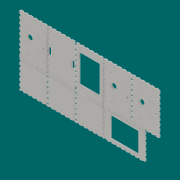
# Autodesk Inventor part: sheetA
Saved by Autodesk Inventor 2016 SP2 (Build 200236200, 236)
## iProperties
Created: 2016-09-27
Part Number: sheetA
Material: Generic
Document SubType Name: Modeling
Designer: sawaiz
Density: 1 g/cm^3
Appearance: Default
Author: sawaiz
Autodesk Inventor part; units mm, degrees
(part 1 of 3)
ref_plane "YZ Plane" through (0, 0, 0) normal (1, 0, 0) x (0, 1, 0)
ref_plane "XZ Plane" through (0, 0, 0) normal (0, 1, 0) x (-1, 0, 0)
sketch "Sketch1" plane through (0, 0, 0) normal (0, 0, 1) x (1, 0, 0)
  circle A0 centre (52.276, -59.1479) radius 1.078 projected
  circle A1 centre (17.276, -59.1479) radius 1.078 projected
  line L0 (43.815, -13.335) -> (40.005, -13.335) projected
  line L1 (40.005, -13.335) -> (40.005, -1.905) projected
  line L2 (40.005, -1.905) -> (43.815, -1.905) projected
  line L3 (43.815, -1.905) -> (43.815, -13.335) projected
  circle A2 centre (38.1, -15.24) radius 1.078 projected
  circle A3 centre (45.72, 0) radius 1.078 projected
  circle A4 centre (45.72, -15.24) radius 1.078 projected
  circle A5 centre (38.1, 0) radius 1.078 projected
  line L4 (54.825, -48.5) -> (56.825, -48.5) projected
  line L5 (56.825, -48.5) -> (56.825, -45) projected
  line L6 (56.825, -45) -> (60, -45) projected
  line L7 (60, -45) -> (60, -35) projected
  line L8 (60, -35) -> (56.825, -35) projected
  line L9 (56.825, -35) -> (56.825, -25) projected
  line L10 (56.825, -25) -> (60, -25) projected
  line L11 (60, -25) -> (60, -15) projected
  line L12 (60, -15) -> (56.825, -15) projected
  line L13 (56.825, -15) -> (56.825, -5) projected
  line L14 (56.825, -5) -> (60, -5) projected
  line L15 (60, -5) -> (60, 5) projected
  line L16 (60, 5) -> (56.825, 5) projected
  line L17 (56.825, 5) -> (56.825, 15) projected
  line L18 (56.825, 15) -> (60, 15) projected
  line L19 (60, 15) -> (60, 25) projected
  line L20 (60, 25) -> (56.825, 25) projected
  line L21 (56.825, 25) -> (56.825, 35) projected
  line L22 (56.825, 35) -> (60, 35) projected
  line L23 (60, 35) -> (60, 45) projected
  line L24 (60, 45) -> (56.825, 45) projected
  line L25 (56.825, 45) -> (56.825, 48.5) projected
  line L26 (56.825, 48.5) -> (54.825, 48.5) projected
  line L27 (54.825, 48.5) -> (54.825, 47.25) projected
  line L28 (54.825, 47.25) -> (52.325, 47.25) projected
  line L29 (52.325, 47.25) -> (52.325, 48.5) projected
  line L30 (52.325, 48.5) -> (46, 48.5) projected
  line L31 (46, 48.5) -> (46, 51.5) projected
  line L32 (46, 51.5) -> (52.325, 51.5) projected
  line L33 (52.325, 51.5) -> (52.325, 52.75) projected
  line L34 (52.325, 52.75) -> (54.825, 52.75) projected
  line L35 (54.825, 52.75) -> (54.825, 51.5) projected
  line L36 (54.825, 51.5) -> (56.825, 51.5) projected
  line L37 (56.825, 51.5) -> (56.825, 55) projected
  line L38 (56.825, 55) -> (60, 55) projected
  line L39 (60, 55) -> (60, 65) projected
  line L40 (60, 65) -> (56.825, 65) projected
  line L41 (56.825, 65) -> (56.825, 75) projected
  line L42 (56.825, 75) -> (60, 75) projected
  line L43 (60, 75) -> (60, 86.825) projected
  line L44 (55, 86.825) -> (60, 86.825) projected
  line L45 (55, 90) -> (55, 86.825) projected
  line L46 (45, 90) -> (55, 90) projected
  line L47 (45, 86.825) -> (45, 90) projected
  line L48 (45, 86.825) -> (35, 86.825) projected
  line L49 (35, 90) -> (35, 86.825) projected
  line L50 (25, 90) -> (35, 90) projected
  line L51 (25, 86.825) -> (25, 90) projected
  line L52 (25, 86.825) -> (15, 86.825) projected
  line L53 (15, 90) -> (15, 86.825) projected
  line L54 (5, 90) -> (15, 90) projected
  line L55 (5, 86.825) -> (5, 90) projected
  line L56 (5, 86.825) -> (-5, 86.825) projected
  line L57 (-5, 90) -> (-5, 86.825) projected
  line L58 (-15, 90) -> (-5, 90) projected
  line L59 (-15, 86.825) -> (-15, 90) projected
  line L60 (-15, 86.825) -> (-25, 86.825) projected
  line L61 (-25, 90) -> (-25, 86.825) projected
  line L62 (-35, 90) -> (-25, 90) projected
  line L63 (-35, 86.825) -> (-35, 90) projected
  line L64 (-35, 86.825) -> (-45, 86.825) projected
  line L65 (-45, 90) -> (-45, 86.825) projected
  line L66 (-55, 90) -> (-45, 90) projected
  line L67 (-55, 86.825) -> (-55, 90) projected
  line L68 (-55, 86.825) -> (-60, 86.825) projected
  line L69 (-60, 75) -> (-60, 86.825) projected
  line L70 (-56.825, 75) -> (-60, 75) projected
  line L71 (-56.825, 75) -> (-56.825, 65) projected
  line L72 (-60, 65) -> (-56.825, 65) projected
  line L73 (-60, 55) -> (-60, 65) projected
  line L74 (-56.825, 55) -> (-60, 55) projected
  line L75 (-56.825, 55) -> (-56.825, 45) projected
  line L76 (-60, 45) -> (-56.825, 45) projected
  line L77 (-60, 35) -> (-60, 45) projected
  line L78 (-56.825, 35) -> (-60, 35) projected
  line L79 (-56.825, 35) -> (-56.825, 25) projected
  line L80 (-60, 25) -> (-56.825, 25) projected
  line L81 (-60, 15) -> (-60, 25) projected
  line L82 (-56.825, 15) -> (-60, 15) projected
  line L83 (-56.825, 15) -> (-56.825, 5) projected
  line L84 (-60, 5) -> (-56.825, 5) projected
  line L85 (-60, -5) -> (-60, 5) projected
  line L86 (-56.825, -5) -> (-60, -5) projected
  line L87 (-56.825, -5) -> (-56.825, -15) projected
  line L88 (-60, -15) -> (-56.825, -15) projected
  line L89 (-60, -25) -> (-60, -15) projected
  line L90 (-56.825, -25) -> (-60, -25) projected
  line L91 (-56.825, -25) -> (-56.825, -35) projected
  line L92 (-60, -35) -> (-56.825, -35) projected
  line L93 (-60, -45) -> (-60, -35) projected
  line L94 (-56.825, -45) -> (-60, -45) projected
  line L95 (-56.825, -45) -> (-56.825, -55) projected
  line L96 (-60, -55) -> (-56.825, -55) projected
  line L97 (-60, -65) -> (-60, -55) projected
  line L98 (-56.825, -65) -> (-60, -65) projected
  line L99 (-56.825, -65) -> (-56.825, -75) projected
  line L100 (-60, -75) -> (-56.825, -75) projected
  line L101 (-60, -75) -> (-60, -86.825) projected
  line L102 (-60, -86.825) -> (-55, -86.825) projected
  line L103 (-55, -86.825) -> (-55, -90) projected
  line L104 (-55, -90) -> (-45, -90) projected
  line L105 (-45, -90) -> (-45, -86.825) projected
  line L106 (-45, -86.825) -> (-35, -86.825) projected
  line L107 (-35, -86.825) -> (-35, -90) projected
  line L108 (-35, -90) -> (-25, -90) projected
  line L109 (-25, -90) -> (-25, -86.825) projected
  line L110 (-25, -86.825) -> (-15, -86.825) projected
  line L111 (-15, -86.825) -> (-15, -90) projected
  line L112 (-15, -90) -> (-5, -90) projected
  line L113 (-5, -90) -> (-5, -86.825) projected
  line L114 (-5, -86.825) -> (5, -86.825) projected
  line L115 (5, -86.825) -> (5, -90) projected
  line L116 (5, -90) -> (15, -90) projected
  line L117 (15, -90) -> (15, -86.825) projected
  line L118 (15, -86.825) -> (25, -86.825) projected
  line L119 (25, -86.825) -> (25, -90) projected
  line L120 (25, -90) -> (35, -90) projected
  line L121 (35, -90) -> (35, -86.825) projected
  line L122 (35, -86.825) -> (45, -86.825) projected
  line L123 (45, -86.825) -> (45, -90) projected
  line L124 (45, -90) -> (55, -90) projected
  line L125 (55, -90) -> (55, -86.825) projected
  line L126 (55, -86.825) -> (60, -86.825) projected
  line L127 (60, -86.825) -> (60, -75) projected
  line L128 (60, -75) -> (56.825, -75) projected
  line L129 (56.825, -75) -> (56.825, -65) projected
  line L130 (56.825, -65) -> (60, -65) projected
  line L131 (60, -65) -> (60, -55) projected
  line L132 (60, -55) -> (56.825, -55) projected
  line L133 (56.825, -55) -> (56.825, -51.5) projected
  line L134 (56.825, -51.5) -> (54.825, -51.5) projected
  line L135 (54.825, -51.5) -> (54.825, -52.75) projected
  line L136 (54.825, -52.75) -> (52.325, -52.75) projected
  line L137 (52.325, -52.75) -> (52.325, -51.5) projected
  line L138 (52.325, -51.5) -> (46, -51.5) projected
  line L139 (46, -51.5) -> (46, -48.5) projected
  line L140 (46, -48.5) -> (52.325, -48.5) projected
  line L141 (52.325, -48.5) -> (52.325, -47.25) projected
  line L142 (52.325, -47.25) -> (54.825, -47.25) projected
  line L143 (54.825, -47.25) -> (54.825, -48.5) projected
  circle A6 centre (22.9972, -27.4451) radius 3 projected
  circle A7 centre (-22.9972, 54) radius 3 projected
  circle A8 centre (22.9972, 27.4451) radius 3 projected
  circle A9 centre (-22.9972, -54) radius 3 projected
  circle A10 centre (-15, 8.175) radius 11 projected
  line L144 (55, -207.185) -> (55, -210.36) projected
  line L145 (55, -210.36) -> (60, -210.36) projected
  line L146 (60, -210.36) -> (60, -205.36) projected
  line L147 (60, -205.36) -> (56.825, -205.36) projected
  line L148 (56.825, -205.36) -> (56.825, -195.36) projected
  line L149 (56.825, -195.36) -> (60, -195.36) projected
  line L150 (60, -195.36) -> (60, -185.36) projected
  line L151 (60, -185.36) -> (56.825, -185.36) projected
  line L152 (56.825, -185.36) -> (56.825, -175.36) projected
  line L153 (56.825, -175.36) -> (60, -175.36) projected
  line L154 (60, -175.36) -> (60, -165.36) projected
  line L155 (60, -165.36) -> (56.825, -165.36) projected
  line L156 (56.825, -165.36) -> (56.825, -155.36) projected
  line L157 (56.825, -155.36) -> (60, -155.36) projected
  line L158 (60, -155.36) -> (60, -145.36) projected
  line L159 (60, -145.36) -> (56.825, -145.36) projected
  line L160 (56.825, -145.36) -> (56.825, -135.36) projected
  line L161 (56.825, -135.36) -> (60, -135.36) projected
  line L162 (60, -135.36) -> (60, -125.36) projected
  line L163 (60, -125.36) -> (56.825, -125.36) projected
  line L164 (56.825, -125.36) -> (56.825, -115.36) projected
  line L165 (56.825, -115.36) -> (60, -115.36) projected
  line L166 (60, -115.36) -> (60, -105.36) projected
  line L167 (60, -105.36) -> (56.825, -105.36) projected
  line L168 (56.825, -105.36) -> (56.825, -95.36) projected
  line L169 (56.825, -95.36) -> (60, -95.36) projected
  line L170 (60, -95.36) -> (60, -90.36) projected
  line L171 (60, -90.36) -> (55, -90.36) projected
  line L172 (55, -90.36) -> (55, -93.535) projected
  line L173 (55, -93.535) -> (45, -93.535) projected
  line L174 (45, -93.535) -> (45, -90.36) projected
  line L175 (45, -90.36) -> (35, -90.36) projected
  line L176 (35, -90.36) -> (35, -93.535) projected
  line L177 (35, -93.535) -> (25, -93.535) projected
  line L178 (25, -93.535) -> (25, -90.36) projected
  line L179 (25, -90.36) -> (15, -90.36) projected
  line L180 (15, -90.36) -> (15, -93.535) projected
  line L181 (15, -93.535) -> (5, -93.535) projected
  line L182 (5, -93.535) -> (5, -90.36) projected
  line L183 (5, -90.36) -> (-5, -90.36) projected
  line L184 (-5, -90.36) -> (-5, -93.535) projected
  line L185 (-5, -93.535) -> (-15, -93.535) projected
  line L186 (-15, -93.535) -> (-15, -90.36) projected
  line L187 (-15, -90.36) -> (-25, -90.36) projected
  line L188 (-25, -90.36) -> (-25, -93.535) projected
  line L189 (-25, -93.535) -> (-35, -93.535) projected
  line L190 (-35, -93.535) -> (-35, -90.36) projected
  line L191 (-35, -90.36) -> (-45, -90.36) projected
  line L192 (-45, -90.36) -> (-45, -93.535) projected
  line L193 (-45, -93.535) -> (-55, -93.535) projected
  line L194 (-55, -93.535) -> (-55, -90.36) projected
  line L195 (-55, -90.36) -> (-60, -90.36) projected
  line L196 (-60, -90.36) -> (-60, -95.36) projected
  line L197 (-60, -95.36) -> (-56.825, -95.36) projected
  line L198 (-56.825, -95.36) -> (-56.825, -105.36) projected
  line L199 (-56.825, -105.36) -> (-60, -105.36) projected
  line L200 (-60, -105.36) -> (-60, -115.36) projected
  line L201 (-60, -115.36) -> (-56.825, -115.36) projected
  line L202 (-56.825, -115.36) -> (-56.825, -125.36) projected
  line L203 (-56.825, -125.36) -> (-60, -125.36) projected
  line L204 (-60, -125.36) -> (-60, -135.36) projected
  line L205 (-60, -135.36) -> (-56.825, -135.36) projected
  line L206 (-56.825, -135.36) -> (-56.825, -145.36) projected
  line L207 (-56.825, -145.36) -> (-60, -145.36) projected
  line L208 (-60, -145.36) -> (-60, -155.36) projected
  line L209 (-60, -155.36) -> (-56.825, -155.36) projected
  line L210 (-56.825, -155.36) -> (-56.825, -165.36) projected
  line L211 (-56.825, -165.36) -> (-60, -165.36) projected
  line L212 (-60, -165.36) -> (-60, -175.36) projected
  line L213 (-60, -175.36) -> (-56.825, -175.36) projected
  line L214 (-56.825, -175.36) -> (-56.825, -185.36) projected
  line L215 (-56.825, -185.36) -> (-60, -185.36) projected
  line L216 (-60, -185.36) -> (-60, -195.36) projected
  line L217 (-60, -195.36) -> (-56.825, -195.36) projected
  line L218 (-56.825, -195.36) -> (-56.825, -205.36) projected
  line L219 (-56.825, -205.36) -> (-60, -205.36) projected
  line L220 (-60, -205.36) -> (-60, -210.36) projected
  line L221 (-60, -210.36) -> (-55, -210.36) projected
  line L222 (-55, -210.36) -> (-55, -207.185) projected
  line L223 (-55, -207.185) -> (-45, -207.185) projected
  line L224 (-45, -207.185) -> (-45, -210.36) projected
  line L225 (-45, -210.36) -> (-35, -210.36) projected
  line L226 (-35, -210.36) -> (-35, -207.185) projected
  line L227 (-35, -207.185) -> (-25, -207.185) projected
  line L228 (-25, -207.185) -> (-25, -210.36) projected
  line L229 (-25, -210.36) -> (-15, -210.36) projected
  line L230 (-15, -210.36) -> (-15, -207.185) projected
  line L231 (-15, -207.185) -> (-5, -207.185) projected
  line L232 (-5, -207.185) -> (-5, -210.36) projected
  line L233 (-5, -210.36) -> (5, -210.36) projected
  line L234 (5, -210.36) -> (5, -207.185) projected
  line L235 (5, -207.185) -> (15, -207.185) projected
  line L236 (15, -207.185) -> (15, -210.36) projected
  line L237 (15, -210.36) -> (25, -210.36) projected
  line L238 (25, -210.36) -> (25, -207.185) projected
  line L239 (25, -207.185) -> (35, -207.185) projected
  line L240 (35, -207.185) -> (35, -210.36) projected
  line L241 (35, -210.36) -> (45, -210.36) projected
  line L242 (45, -210.36) -> (45, -207.185) projected
  line L243 (45, -207.185) -> (55, -207.185) projected
  line L244 (175.36, -207.185) -> (175.36, -210.36) projected
  line L245 (175.36, -210.36) -> (180.36, -210.36) projected
  line L246 (180.36, -210.36) -> (180.36, -205.36) projected
  line L247 (180.36, -205.36) -> (177.185, -205.36) projected
  line L248 (177.185, -205.36) -> (177.185, -195.36) projected
  line L249 (177.185, -195.36) -> (180.36, -195.36) projected
  line L250 (180.36, -195.36) -> (180.36, -185.36) projected
  line L251 (180.36, -185.36) -> (177.185, -185.36) projected
  line L252 (177.185, -185.36) -> (177.185, -175.36) projected
  line L253 (177.185, -175.36) -> (180.36, -175.36) projected
  line L254 (180.36, -175.36) -> (180.36, -165.36) projected
  line L255 (180.36, -165.36) -> (177.185, -165.36) projected
  line L256 (177.185, -165.36) -> (177.185, -155.36) projected
  line L257 (177.185, -155.36) -> (180.36, -155.36) projected
  line L258 (180.36, -155.36) -> (180.36, -145.36) projected
  line L259 (180.36, -145.36) -> (177.185, -145.36) projected
  line L260 (177.185, -145.36) -> (177.185, -135.36) projected
  line L261 (177.185, -135.36) -> (180.36, -135.36) projected
  line L262 (180.36, -135.36) -> (180.36, -125.36) projected
  line L263 (180.36, -125.36) -> (177.185, -125.36) projected
  line L264 (177.185, -125.36) -> (177.185, -115.36) projected
  line L265 (177.185, -115.36) -> (180.36, -115.36) projected
  line L266 (180.36, -115.36) -> (180.36, -105.36) projected
  line L267 (180.36, -105.36) -> (177.185, -105.36) projected
  line L268 (177.185, -105.36) -> (177.185, -95.36) projected
  line L269 (177.185, -95.36) -> (180.36, -95.36) projected
  line L270 (180.36, -95.36) -> (180.36, -90.36) projected
  line L271 (180.36, -90.36) -> (175.36, -90.36) projected
  line L272 (175.36, -90.36) -> (175.36, -93.535) projected
  line L273 (175.36, -93.535) -> (165.36, -93.535) projected
  line L274 (165.36, -93.535) -> (165.36, -90.36) projected
  line L275 (165.36, -90.36) -> (155.36, -90.36) projected
  line L276 (155.36, -90.36) -> (155.36, -93.535) projected
  line L277 (155.36, -93.535) -> (145.36, -93.535) projected
  line L278 (145.36, -93.535) -> (145.36, -90.36) projected
  line L279 (145.36, -90.36) -> (135.36, -90.36) projected
  line L280 (135.36, -90.36) -> (135.36, -93.535) projected
  line L281 (135.36, -93.535) -> (125.36, -93.535) projected
  line L282 (125.36, -93.535) -> (125.36, -90.36) projected
  line L283 (125.36, -90.36) -> (115.36, -90.36) projected
  line L284 (115.36, -90.36) -> (115.36, -93.535) projected
  line L285 (115.36, -93.535) -> (105.36, -93.535) projected
  line L286 (105.36, -93.535) -> (105.36, -90.36) projected
  line L287 (105.36, -90.36) -> (95.36, -90.36) projected
  line L288 (95.36, -90.36) -> (95.36, -93.535) projected
  line L289 (95.36, -93.535) -> (85.36, -93.535) projected
  line L290 (85.36, -93.535) -> (85.36, -90.36) projected
  line L291 (85.36, -90.36) -> (75.36, -90.36) projected
  line L292 (75.36, -90.36) -> (75.36, -93.535) projected
  line L293 (75.36, -93.535) -> (65.36, -93.535) projected
  line L294 (65.36, -93.535) -> (65.36, -90.36) projected
  line L295 (65.36, -90.36) -> (60.36, -90.36) projected
  line L296 (60.36, -90.36) -> (60.36, -95.36) projected
  line L297 (60.36, -95.36) -> (63.535, -95.36) projected
  line L298 (63.535, -95.36) -> (63.535, -105.36) projected
  line L299 (63.535, -105.36) -> (60.36, -105.36) projected
  line L300 (60.36, -105.36) -> (60.36, -115.36) projected
  line L301 (60.36, -115.36) -> (63.535, -115.36) projected
  line L302 (63.535, -115.36) -> (63.535, -125.36) projected
  line L303 (63.535, -125.36) -> (60.36, -125.36) projected
  line L304 (60.36, -125.36) -> (60.36, -135.36) projected
  line L305 (60.36, -135.36) -> (63.535, -135.36) projected
  line L306 (63.535, -135.36) -> (63.535, -145.36) projected
  line L307 (63.535, -145.36) -> (60.36, -145.36) projected
  line L308 (60.36, -145.36) -> (60.36, -155.36) projected
  line L309 (60.36, -155.36) -> (63.535, -155.36) projected
  line L310 (63.535, -155.36) -> (63.535, -165.36) projected
  line L311 (63.535, -165.36) -> (60.36, -165.36) projected
  line L312 (60.36, -165.36) -> (60.36, -175.36) projected
  line L313 (60.36, -175.36) -> (63.535, -175.36) projected
  line L314 (63.535, -175.36) -> (63.535, -185.36) projected
  line L315 (63.535, -185.36) -> (60.36, -185.36) projected
  line L316 (60.36, -185.36) -> (60.36, -195.36) projected
  line L317 (60.36, -195.36) -> (63.535, -195.36) projected
  line L318 (63.535, -195.36) -> (63.535, -205.36) projected
  line L319 (63.535, -205.36) -> (60.36, -205.36) projected
  line L320 (60.36, -205.36) -> (60.36, -210.36) projected
  line L321 (60.36, -210.36) -> (65.36, -210.36) projected
  line L322 (65.36, -210.36) -> (65.36, -207.185) projected
  line L323 (65.36, -207.185) -> (75.36, -207.185) projected
  line L324 (75.36, -207.185) -> (75.36, -210.36) projected
  line L325 (75.36, -210.36) -> (85.36, -210.36) projected
  line L326 (85.36, -210.36) -> (85.36, -207.185) projected
  line L327 (85.36, -207.185) -> (95.36, -207.185) projected
  line L328 (95.36, -207.185) -> (95.36, -210.36) projected
  line L329 (95.36, -210.36) -> (105.36, -210.36) projected
  line L330 (105.36, -210.36) -> (105.36, -207.185) projected
  line L331 (105.36, -207.185) -> (115.36, -207.185) projected
  line L332 (115.36, -207.185) -> (115.36, -210.36) projected
  line L333 (115.36, -210.36) -> (125.36, -210.36) projected
  line L334 (125.36, -210.36) -> (125.36, -207.185) projected
  line L335 (125.36, -207.185) -> (135.36, -207.185) projected
  line L336 (135.36, -207.185) -> (135.36, -210.36) projected
  line L337 (135.36, -210.36) -> (145.36, -210.36) projected
  line L338 (145.36, -210.36) -> (145.36, -207.185) projected
  line L339 (145.36, -207.185) -> (155.36, -207.185) projected
  line L340 (155.36, -207.185) -> (155.36, -210.36) projected
  line L341 (155.36, -210.36) -> (165.36, -210.36) projected
  line L342 (165.36, -210.36) -> (165.36, -207.185) projected
  line L343 (165.36, -207.185) -> (175.36, -207.185) projected
  line L344 (165.36, -15) -> (165.36, 15) projected
  line L345 (165.36, 15) -> (175.36, 15) projected
  line L346 (175.36, 15) -> (175.36, -15) projected
  line L347 (175.36, -15) -> (165.36, -15) projected
  line L348 (65.36, -15) -> (65.36, 15) projected
  line L349 (65.36, 15) -> (75.36, 15) projected
  line L350 (75.36, 15) -> (75.36, -15) projected
  line L351 (75.36, -15) -> (65.36, -15) projected
  circle A11 centre (177.185, -50) radius 1.7 projected
  circle A12 centre (177.185, 50) radius 1.7 projected
  circle A13 centre (63.535, -50) radius 1.7 projected
  circle A14 centre (63.535, 50) radius 1.7 projected
  line L352 (177.185, 75) -> (177.185, 86.825) projected
  line L353 (177.185, 86.825) -> (175.36, 86.825) projected
  line L354 (175.36, 86.825) -> (175.36, 90) projected
  line L355 (175.36, 90) -> (165.36, 90) projected
  line L356 (165.36, 90) -> (165.36, 86.825) projected
  line L357 (165.36, 86.825) -> (155.36, 86.825) projected
  line L358 (155.36, 86.825) -> (155.36, 90) projected
  line L359 (155.36, 90) -> (145.36, 90) projected
  line L360 (145.36, 90) -> (145.36, 86.825) projected
  line L361 (145.36, 86.825) -> (135.36, 86.825) projected
  line L362 (135.36, 86.825) -> (135.36, 90) projected
  line L363 (135.36, 90) -> (125.36, 90) projected
  line L364 (125.36, 90) -> (125.36, 86.825) projected
  line L365 (125.36, 86.825) -> (115.36, 86.825) projected
  line L366 (115.36, 86.825) -> (115.36, 90) projected
  line L367 (115.36, 90) -> (105.36, 90) projected
  line L368 (105.36, 90) -> (105.36, 86.825) projected
  line L369 (105.36, 86.825) -> (95.36, 86.825) projected
  line L370 (95.36, 86.825) -> (95.36, 90) projected
  line L371 (95.36, 90) -> (85.36, 90) projected
  line L372 (85.36, 90) -> (85.36, 86.825) projected
  line L373 (85.36, 86.825) -> (75.36, 86.825) projected
  line L374 (75.36, 86.825) -> (75.36, 90) projected
  line L375 (75.36, 90) -> (65.36, 90) projected
  line L376 (65.36, 90) -> (65.36, 86.825) projected
  line L377 (65.36, 86.825) -> (63.535, 86.825) projected
  line L378 (63.535, 86.825) -> (63.535, 75) projected
  line L379 (63.535, 75) -> (60.36, 75) projected
  line L380 (60.36, 75) -> (60.36, 65) projected
  line L381 (60.36, 65) -> (63.535, 65) projected
  line L382 (63.535, 65) -> (63.535, 55) projected
  line L383 (63.535, 55) -> (60.36, 55) projected
  line L384 (60.36, 55) -> (60.36, 45) projected
  line L385 (60.36, 45) -> (63.535, 45) projected
  line L386 (63.535, 45) -> (63.535, 35) projected
  line L387 (63.535, 35) -> (60.36, 35) projected
  line L388 (60.36, 35) -> (60.36, 25) projected
  line L389 (60.36, 25) -> (63.535, 25) projected
  line L390 (63.535, 25) -> (63.535, 15) projected
  line L391 (63.535, 15) -> (60.36, 15) projected
  line L392 (60.36, 15) -> (60.36, 5) projected
  line L393 (60.36, 5) -> (63.535, 5) projected
  line L394 (63.535, 5) -> (63.535, -5) projected
  line L395 (63.535, -5) -> (60.36, -5) projected
  line L396 (60.36, -5) -> (60.36, -15) projected
  line L397 (60.36, -15) -> (63.535, -15) projected
  line L398 (63.535, -15) -> (63.535, -25) projected
  line L399 (63.535, -25) -> (60.36, -25) projected
  line L400 (60.36, -25) -> (60.36, -35) projected
  line L401 (60.36, -35) -> (63.535, -35) projected
  line L402 (63.535, -35) -> (63.535, -45) projected
  line L403 (63.535, -45) -> (60.36, -45) projected
  line L404 (60.36, -45) -> (60.36, -55) projected
  line L405 (60.36, -55) -> (63.535, -55) projected
  line L406 (63.535, -55) -> (63.535, -65) projected
  line L407 (63.535, -65) -> (60.36, -65) projected
  line L408 (60.36, -65) -> (60.36, -75) projected
  line L409 (60.36, -75) -> (63.535, -75) projected
  line L410 (63.535, -75) -> (63.535, -86.825) projected
  line L411 (63.535, -86.825) -> (65.36, -86.825) projected
  line L412 (65.36, -86.825) -> (65.36, -90) projected
  line L413 (65.36, -90) -> (75.36, -90) projected
  line L414 (75.36, -90) -> (75.36, -86.825) projected
  line L415 (75.36, -86.825) -> (85.36, -86.825) projected
  line L416 (85.36, -86.825) -> (85.36, -90) projected
  line L417 (85.36, -90) -> (95.36, -90) projected
  line L418 (95.36, -90) -> (95.36, -86.825) projected
  line L419 (95.36, -86.825) -> (105.36, -86.825) projected
  line L420 (105.36, -86.825) -> (105.36, -90) projected
  line L421 (105.36, -90) -> (115.36, -90) projected
  line L422 (115.36, -90) -> (115.36, -86.825) projected
  line L423 (115.36, -86.825) -> (125.36, -86.825) projected
  line L424 (125.36, -86.825) -> (125.36, -90) projected
  line L425 (125.36, -90) -> (135.36, -90) projected
  line L426 (135.36, -90) -> (135.36, -86.825) projected
  line L427 (135.36, -86.825) -> (145.36, -86.825) projected
  line L428 (145.36, -86.825) -> (145.36, -90) projected
  line L429 (145.36, -90) -> (155.36, -90) projected
  line L430 (155.36, -90) -> (155.36, -86.825) projected
  line L431 (155.36, -86.825) -> (165.36, -86.825) projected
  line L432 (165.36, -86.825) -> (165.36, -90) projected
  line L433 (165.36, -90) -> (175.36, -90) projected
  line L434 (175.36, -90) -> (175.36, -86.825) projected
  line L435 (175.36, -86.825) -> (177.185, -86.825) projected
  line L436 (177.185, -86.825) -> (177.185, -75) projected
  line L437 (177.185, -75) -> (180.36, -75) projected
  line L438 (180.36, -75) -> (180.36, -65) projected
  line L439 (180.36, -65) -> (177.185, -65) projected
  line L440 (177.185, -65) -> (177.185, -55) projected
  line L441 (177.185, -55) -> (180.36, -55) projected
  line L442 (180.36, -55) -> (180.36, -45) projected
  line L443 (180.36, -45) -> (177.185, -45) projected
  line L444 (177.185, -45) -> (177.185, -35) projected
  line L445 (177.185, -35) -> (180.36, -35) projected
  line L446 (180.36, -35) -> (180.36, -25) projected
  line L447 (180.36, -25) -> (177.185, -25) projected
  line L448 (177.185, -25) -> (177.185, -15) projected
  line L449 (177.185, -15) -> (180.36, -15) projected
  line L450 (180.36, -15) -> (180.36, -5) projected
  line L451 (180.36, -5) -> (177.185, -5) projected
  line L452 (177.185, -5) -> (177.185, 5) projected
  line L453 (177.185, 5) -> (180.36, 5) projected
  line L454 (180.36, 5) -> (180.36, 15) projected
  line L455 (180.36, 15) -> (177.185, 15) projected
  line L456 (177.185, 15) -> (177.185, 25) projected
  line L457 (177.185, 25) -> (180.36, 25) projected
  line L458 (180.36, 25) -> (180.36, 35) projected
  line L459 (180.36, 35) -> (177.185, 35) projected
  line L460 (177.185, 35) -> (177.185, 45) projected
  line L461 (177.185, 45) -> (180.36, 45) projected
  line L462 (180.36, 45) -> (180.36, 55) projected
  line L463 (180.36, 55) -> (177.185, 55) projected
  line L464 (177.185, 55) -> (177.185, 65) projected
  line L465 (177.185, 65) -> (180.36, 65) projected
  line L466 (180.36, 65) -> (180.36, 75) projected
  line L467 (180.36, 75) -> (177.185, 75) projected
  line L468 (295.72, -207.185) -> (295.72, -210.36) projected
  line L469 (295.72, -210.36) -> (300.72, -210.36) projected
  line L470 (300.72, -210.36) -> (300.72, -205.36) projected
  line L471 (300.72, -205.36) -> (297.545, -205.36) projected
  line L472 (297.545, -205.36) -> (297.545, -195.36) projected
  line L473 (297.545, -195.36) -> (300.72, -195.36) projected
  line L474 (300.72, -195.36) -> (300.72, -185.36) projected
  line L475 (300.72, -185.36) -> (297.545, -185.36) projected
  line L476 (297.545, -185.36) -> (297.545, -175.36) projected
  line L477 (297.545, -175.36) -> (300.72, -175.36) projected
  line L478 (300.72, -175.36) -> (300.72, -165.36) projected
  line L479 (300.72, -165.36) -> (297.545, -165.36) projected
  line L480 (297.545, -165.36) -> (297.545, -155.36) projected
  line L481 (297.545, -155.36) -> (300.72, -155.36) projected
  line L482 (300.72, -155.36) -> (300.72, -145.36) projected
  line L483 (300.72, -145.36) -> (297.545, -145.36) projected
  line L484 (297.545, -145.36) -> (297.545, -135.36) projected
  line L485 (297.545, -135.36) -> (300.72, -135.36) projected
  line L486 (300.72, -135.36) -> (300.72, -125.36) projected
  line L487 (300.72, -125.36) -> (297.545, -125.36) projected
  line L488 (297.545, -125.36) -> (297.545, -115.36) projected
  line L489 (297.545, -115.36) -> (300.72, -115.36) projected
  line L490 (300.72, -115.36) -> (300.72, -105.36) projected
  line L491 (300.72, -105.36) -> (297.545, -105.36) projected
  line L492 (297.545, -105.36) -> (297.545, -95.36) projected
  line L493 (297.545, -95.36) -> (300.72, -95.36) projected
  line L494 (300.72, -95.36) -> (300.72, -90.36) projected
  line L495 (300.72, -90.36) -> (295.72, -90.36) projected
  line L496 (295.72, -90.36) -> (295.72, -93.535) projected
  line L497 (295.72, -93.535) -> (285.72, -93.535) projected
  line L498 (285.72, -93.535) -> (285.72, -90.36) projected
  line L499 (285.72, -90.36) -> (275.72, -90.36) projected
  line L500 (275.72, -90.36) -> (275.72, -93.535) projected
  line L501 (275.72, -93.535) -> (265.72, -93.535) projected
  line L502 (265.72, -93.535) -> (265.72, -90.36) projected
  line L503 (265.72, -90.36) -> (255.72, -90.36) projected
  line L504 (255.72, -90.36) -> (255.72, -93.535) projected
  line L505 (255.72, -93.535) -> (245.72, -93.535) projected
  line L506 (245.72, -93.535) -> (245.72, -90.36) projected
  line L507 (245.72, -90.36) -> (235.72, -90.36) projected
  line L508 (235.72, -90.36) -> (235.72, -93.535) projected
  line L509 (235.72, -93.535) -> (225.72, -93.535) projected
  line L510 (225.72, -93.535) -> (225.72, -90.36) projected
  line L511 (225.72, -90.36) -> (215.72, -90.36) projected
  line L512 (215.72, -90.36) -> (215.72, -93.535) projected
  line L513 (215.72, -93.535) -> (205.72, -93.535) projected
  line L514 (205.72, -93.535) -> (205.72, -90.36) projected
  line L515 (205.72, -90.36) -> (195.72, -90.36) projected
  line L516 (195.72, -90.36) -> (195.72, -93.535) projected
  line L517 (195.72, -93.535) -> (185.72, -93.535) projected
  line L518 (185.72, -93.535) -> (185.72, -90.36) projected
  line L519 (185.72, -90.36) -> (180.72, -90.36) projected
  line L520 (180.72, -90.36) -> (180.72, -95.36) projected
  line L521 (180.72, -95.36) -> (183.895, -95.36) projected
  line L522 (183.895, -95.36) -> (183.895, -105.36) projected
  line L523 (183.895, -105.36) -> (180.72, -105.36) projected
  line L524 (180.72, -105.36) -> (180.72, -115.36) projected
  line L525 (180.72, -115.36) -> (183.895, -115.36) projected
  line L526 (183.895, -115.36) -> (183.895, -125.36) projected
  line L527 (183.895, -125.36) -> (180.72, -125.36) projected
  line L528 (180.72, -125.36) -> (180.72, -135.36) projected
  line L529 (180.72, -135.36) -> (183.895, -135.36) projected
  line L530 (183.895, -135.36) -> (183.895, -145.36) projected
  line L531 (183.895, -145.36) -> (180.72, -145.36) projected
  line L532 (180.72, -145.36) -> (180.72, -155.36) projected
  line L533 (180.72, -155.36) -> (183.895, -155.36) projected
  line L534 (183.895, -155.36) -> (183.895, -165.36) projected
  line L535 (183.895, -165.36) -> (180.72, -165.36) projected
  line L536 (180.72, -165.36) -> (180.72, -175.36) projected
  line L537 (180.72, -175.36) -> (183.895, -175.36) projected
  line L538 (183.895, -175.36) -> (183.895, -185.36) projected
  line L539 (183.895, -185.36) -> (180.72, -185.36) projected
  line L540 (180.72, -185.36) -> (180.72, -195.36) projected
  line L541 (180.72, -195.36) -> (183.895, -195.36) projected
  line L542 (183.895, -195.36) -> (183.895, -205.36) projected
  line L543 (183.895, -205.36) -> (180.72, -205.36) projected
  line L544 (180.72, -205.36) -> (180.72, -210.36) projected
  line L545 (180.72, -210.36) -> (185.72, -210.36) projected
  line L546 (185.72, -210.36) -> (185.72, -207.185) projected
  line L547 (185.72, -207.185) -> (195.72, -207.185) projected
  line L548 (195.72, -207.185) -> (195.72, -210.36) projected
  line L549 (195.72, -210.36) -> (205.72, -210.36) projected
  line L550 (205.72, -210.36) -> (205.72, -207.185) projected
  line L551 (205.72, -207.185) -> (215.72, -207.185) projected
  line L552 (215.72, -207.185) -> (215.72, -210.36) projected
  line L553 (215.72, -210.36) -> (225.72, -210.36) projected
  line L554 (225.72, -210.36) -> (225.72, -207.185) projected
  line L555 (225.72, -207.185) -> (235.72, -207.185) projected
  line L556 (235.72, -207.185) -> (235.72, -210.36) projected
  line L557 (235.72, -210.36) -> (245.72, -210.36) projected
  line L558 (245.72, -210.36) -> (245.72, -207.185) projected
  line L559 (245.72, -207.185) -> (255.72, -207.185) projected
  line L560 (255.72, -207.185) -> (255.72, -210.36) projected
  line L561 (255.72, -210.36) -> (265.72, -210.36) projected
  line L562 (265.72, -210.36) -> (265.72, -207.185) projected
  line L563 (265.72, -207.185) -> (275.72, -207.185) projected
  line L564 (275.72, -207.185) -> (275.72, -210.36) projected
  line L565 (275.72, -210.36) -> (285.72, -210.36) projected
  line L566 (285.72, -210.36) -> (285.72, -207.185) projected
  line L567 (285.72, -207.185) -> (295.72, -207.185) projected
  line L568 (297.545, 75) -> (297.545, 86.825) projected
  line L569 (297.545, 86.825) -> (295.72, 86.825) projected
  line L570 (295.72, 86.825) -> (295.72, 90) projected
  line L571 (295.72, 90) -> (285.72, 90) projected
  line L572 (285.72, 90) -> (285.72, 86.825) projected
  line L573 (285.72, 86.825) -> (275.72, 86.825) projected
  line L574 (275.72, 86.825) -> (275.72, 90) projected
  line L575 (275.72, 90) -> (265.72, 90) projected
  line L576 (265.72, 90) -> (265.72, 86.825) projected
  line L577 (265.72, 86.825) -> (255.72, 86.825) projected
  line L578 (255.72, 86.825) -> (255.72, 90) projected
  line L579 (255.72, 90) -> (245.72, 90) projected
  line L580 (245.72, 90) -> (245.72, 86.825) projected
  line L581 (245.72, 86.825) -> (235.72, 86.825) projected
  line L582 (235.72, 86.825) -> (235.72, 90) projected
  line L583 (235.72, 90) -> (225.72, 90) projected
  line L584 (225.72, 90) -> (225.72, 86.825) projected
  line L585 (225.72, 86.825) -> (215.72, 86.825) projected
  line L586 (215.72, 86.825) -> (215.72, 90) projected
  line L587 (215.72, 90) -> (205.72, 90) projected
  line L588 (205.72, 90) -> (205.72, 86.825) projected
  line L589 (205.72, 86.825) -> (195.72, 86.825) projected
  line L590 (195.72, 86.825) -> (195.72, 90) projected
  line L591 (195.72, 90) -> (185.72, 90) projected
  line L592 (185.72, 90) -> (185.72, 86.825) projected
  line L593 (185.72, 86.825) -> (183.895, 86.825) projected
  line L594 (183.895, 86.825) -> (183.895, 75) projected
  line L595 (183.895, 75) -> (180.72, 75) projected
  line L596 (180.72, 75) -> (180.72, 65) projected
  line L597 (180.72, 65) -> (183.895, 65) projected
  line L598 (183.895, 65) -> (183.895, 55) projected
  line L599 (183.895, 55) -> (180.72, 55) projected
  line L600 (180.72, 55) -> (180.72, 45) projected
  line L601 (180.72, 45) -> (183.895, 45) projected
  line L602 (183.895, 45) -> (183.895, 35) projected
  line L603 (183.895, 35) -> (180.72, 35) projected
  line L604 (180.72, 35) -> (180.72, 25) projected
  line L605 (180.72, 25) -> (183.895, 25) projected
  line L606 (183.895, 25) -> (183.895, 15) projected
  line L607 (183.895, 15) -> (180.72, 15) projected
  line L608 (180.72, 15) -> (180.72, 5) projected
  line L609 (180.72, 5) -> (183.895, 5) projected
  line L610 (183.895, 5) -> (183.895, -5) projected
  line L611 (183.895, -5) -> (180.72, -5) projected
  line L612 (180.72, -5) -> (180.72, -15) projected
  line L613 (180.72, -15) -> (183.895, -15) projected
  line L614 (183.895, -15) -> (183.895, -25) projected
  line L615 (183.895, -25) -> (180.72, -25) projected
  line L616 (180.72, -25) -> (180.72, -35) projected
  line L617 (180.72, -35) -> (183.895, -35) projected
  line L618 (183.895, -35) -> (183.895, -45) projected
  line L619 (183.895, -45) -> (180.72, -45) projected
  line L620 (180.72, -45) -> (180.72, -55) projected
  line L621 (180.72, -55) -> (183.895, -55) projected
  line L622 (183.895, -55) -> (183.895, -65) projected
  line L623 (183.895, -65) -> (180.72, -65) projected
  line L624 (180.72, -65) -> (180.72, -75) projected
  line L625 (180.72, -75) -> (183.895, -75) projected
  line L626 (183.895, -75) -> (183.895, -86.825) projected
  line L627 (183.895, -86.825) -> (185.72, -86.825) projected
  line L628 (185.72, -86.825) -> (185.72, -90) projected
  line L629 (185.72, -90) -> (195.72, -90) projected
  line L630 (195.72, -90) -> (195.72, -86.825) projected
  line L631 (195.72, -86.825) -> (205.72, -86.825) projected
  line L632 (205.72, -86.825) -> (205.72, -90) projected
  line L633 (205.72, -90) -> (215.72, -90) projected
  line L634 (215.72, -90) -> (215.72, -86.825) projected
  line L635 (215.72, -86.825) -> (225.72, -86.825) projected
  line L636 (225.72, -86.825) -> (225.72, -90) projected
  line L637 (225.72, -90) -> (235.72, -90) projected
  line L638 (235.72, -90) -> (235.72, -86.825) projected
  line L639 (235.72, -86.825) -> (245.72, -86.825) projected
  line L640 (245.72, -86.825) -> (245.72, -90) projected
  line L641 (245.72, -90) -> (255.72, -90) projected
  line L642 (255.72, -90) -> (255.72, -86.825) projected
  line L643 (255.72, -86.825) -> (265.72, -86.825) projected
  line L644 (265.72, -86.825) -> (265.72, -90) projected
  line L645 (265.72, -90) -> (275.72, -90) projected
  line L646 (275.72, -90) -> (275.72, -86.825) projected
  line L647 (275.72, -86.825) -> (285.72, -86.825) projected
  line L648 (285.72, -86.825) -> (285.72, -90) projected
  line L649 (285.72, -90) -> (295.72, -90) projected
  line L650 (295.72, -90) -> (295.72, -86.825) projected
  line L651 (295.72, -86.825) -> (297.545, -86.825) projected
  line L652 (297.545, -86.825) -> (297.545, -75) projected
  line L653 (297.545, -75) -> (300.72, -75) projected
  line L654 (300.72, -75) -> (300.72, -65) projected
  line L655 (300.72, -65) -> (297.545, -65) projected
  line L656 (297.545, -65) -> (297.545, -55) projected
  line L657 (297.545, -55) -> (300.72, -55) projected
  line L658 (300.72, -55) -> (300.72, -45) projected
  line L659 (300.72, -45) -> (297.545, -45) projected
  line L660 (297.545, -45) -> (297.545, -35) projected
  line L661 (297.545, -35) -> (300.72, -35) projected
  line L662 (300.72, -35) -> (300.72, -25) projected
  line L663 (300.72, -25) -> (297.545, -25) projected
  line L664 (297.545, -25) -> (297.545, -15) projected
  line L665 (297.545, -15) -> (300.72, -15) projected
  line L666 (300.72, -15) -> (300.72, -5) projected
  line L667 (300.72, -5) -> (297.545, -5) projected
  line L668 (297.545, -5) -> (297.545, 5) projected
  line L669 (297.545, 5) -> (300.72, 5) projected
  line L670 (300.72, 5) -> (300.72, 15) projected
  line L671 (300.72, 15) -> (297.545, 15) projected
  line L672 (297.545, 15) -> (297.545, 25) projected
  line L673 (297.545, 25) -> (300.72, 25) projected
  line L674 (300.72, 25) -> (300.72, 35) projected
  line L675 (300.72, 35) -> (297.545, 35) projected
  line L676 (297.545, 35) -> (297.545, 45) projected
  line L677 (297.545, 45) -> (300.72, 45) projected
  line L678 (300.72, 45) -> (300.72, 55) projected
  line L679 (300.72, 55) -> (297.545, 55) projected
  line L680 (297.545, 55) -> (297.545, 65) projected
  line L681 (297.545, 65) -> (300.72, 65) projected
  line L682 (300.72, 65) -> (300.72, 75) projected
  line L683 (300.72, 75) -> (297.545, 75) projected
  line L684 (196.92, -60) -> (196.92, 60) projected
  line L685 (196.92, 60) -> (284.52, 60) projected
  line L686 (284.52, 60) -> (284.52, -60) projected
  line L687 (284.52, -60) -> (196.92, -60) projected
  line L688 (404.895, -13.335) -> (401.085, -13.335) projected
  line L689 (401.085, -13.335) -> (401.085, -1.905) projected
  line L690 (401.085, -1.905) -> (404.895, -1.905) projected
  line L691 (404.895, -1.905) -> (404.895, -13.335) projected
  circle A15 centre (399.18, -15.24) radius 1.078 projected
  circle A16 centre (406.8, 0) radius 1.078 projected
  circle A17 centre (406.8, -15.24) radius 1.078 projected
  circle A18 centre (399.18, 0) radius 1.078 projected
  line L692 (415.905, -48.5) -> (417.905, -48.5) projected
  line L693 (417.905, -48.5) -> (417.905, -45) projected
  line L694 (417.905, -45) -> (421.08, -45) projected
  line L695 (421.08, -45) -> (421.08, -35) projected
  line L696 (421.08, -35) -> (417.905, -35) projected
  line L697 (417.905, -35) -> (417.905, -25) projected
  line L698 (417.905, -25) -> (421.08, -25) projected
  line L699 (421.08, -25) -> (421.08, -15) projected
  line L700 (421.08, -15) -> (417.905, -15) projected
  line L701 (417.905, -15) -> (417.905, -5) projected
  line L702 (417.905, -5) -> (421.08, -5) projected
  line L703 (421.08, -5) -> (421.08, 5) projected
  line L704 (421.08, 5) -> (417.905, 5) projected
  line L705 (417.905, 5) -> (417.905, 15) projected
  line L706 (417.905, 15) -> (421.08, 15) projected
  line L707 (421.08, 15) -> (421.08, 25) projected
  line L708 (421.08, 25) -> (417.905, 25) projected
  line L709 (417.905, 25) -> (417.905, 35) projected
  line L710 (417.905, 35) -> (421.08, 35) projected
  line L711 (421.08, 35) -> (421.08, 45) projected
  line L712 (421.08, 45) -> (417.905, 45) projected
  line L713 (417.905, 45) -> (417.905, 48.5) projected
  line L714 (417.905, 48.5) -> (415.905, 48.5) projected
  line L715 (415.905, 48.5) -> (415.905, 47.25) projected
  line L716 (415.905, 47.25) -> (413.405, 47.25) projected
  line L717 (413.405, 47.25) -> (413.405, 48.5) projected
  line L718 (413.405, 48.5) -> (407.08, 48.5) projected
  line L719 (407.08, 48.5) -> (407.08, 51.5) projected
  line L720 (407.08, 51.5) -> (413.405, 51.5) projected
  line L721 (413.405, 51.5) -> (413.405, 52.75) projected
  line L722 (413.405, 52.75) -> (415.905, 52.75) projected
  line L723 (415.905, 52.75) -> (415.905, 51.5) projected
  line L724 (415.905, 51.5) -> (417.905, 51.5) projected
  line L725 (417.905, 51.5) -> (417.905, 55) projected
  line L726 (417.905, 55) -> (421.08, 55) projected
  line L727 (421.08, 55) -> (421.08, 65) projected
  line L728 (421.08, 65) -> (417.905, 65) projected
  line L729 (417.905, 65) -> (417.905, 75) projected
  line L730 (417.905, 75) -> (421.08, 75) projected
  line L731 (421.08, 75) -> (421.08, 86.825) projected
  line L732 (416.08, 86.825) -> (421.08, 86.825) projected
  line L733 (416.08, 90) -> (416.08, 86.825) projected
  line L734 (406.08, 90) -> (416.08, 90) projected
  line L735 (406.08, 86.825) -> (406.08, 90) projected
  line L736 (406.08, 86.825) -> (396.08, 86.825) projected
  line L737 (396.08, 90) -> (396.08, 86.825) projected
  line L738 (386.08, 90) -> (396.08, 90) projected
  line L739 (386.08, 86.825) -> (386.08, 90) projected
  line L740 (386.08, 86.825) -> (376.08, 86.825) projected
  line L741 (376.08, 90) -> (376.08, 86.825) projected
  line L742 (366.08, 90) -> (376.08, 90) projected
  line L743 (366.08, 86.825) -> (366.08, 90) projected
  line L744 (366.08, 86.825) -> (356.08, 86.825) projected
  line L745 (356.08, 90) -> (356.08, 86.825) projected
  line L746 (346.08, 90) -> (356.08, 90) projected
  line L747 (346.08, 86.825) -> (346.08, 90) projected
  line L748 (346.08, 86.825) -> (336.08, 86.825) projected
  line L749 (336.08, 90) -> (336.08, 86.825) projected
  line L750 (326.08, 90) -> (336.08, 90) projected
  line L751 (326.08, 86.825) -> (326.08, 90) projected
  line L752 (326.08, 86.825) -> (316.08, 86.825) projected
  line L753 (316.08, 90) -> (316.08, 86.825) projected
  line L754 (306.08, 90) -> (316.08, 90) projected
  line L755 (306.08, 86.825) -> (306.08, 90) projected
  line L756 (306.08, 86.825) -> (301.08, 86.825) projected
  line L757 (301.08, 75) -> (301.08, 86.825) projected
  line L758 (304.255, 75) -> (301.08, 75) projected
  line L759 (304.255, 75) -> (304.255, 65) projected
  line L760 (301.08, 65) -> (304.255, 65) projected
  line L761 (301.08, 55) -> (301.08, 65) projected
  line L762 (304.255, 55) -> (301.08, 55) projected
  line L763 (304.255, 55) -> (304.255, 45) projected
  line L764 (301.08, 45) -> (304.255, 45) projected
  line L765 (301.08, 35) -> (301.08, 45) projected
  line L766 (304.255, 35) -> (301.08, 35) projected
  line L767 (304.255, 35) -> (304.255, 25) projected
  line L768 (301.08, 25) -> (304.255, 25) projected
  line L769 (301.08, 15) -> (301.08, 25) projected
  line L770 (304.255, 15) -> (301.08, 15) projected
  line L771 (304.255, 15) -> (304.255, 5) projected
  line L772 (301.08, 5) -> (304.255, 5) projected
  line L773 (301.08, -5) -> (301.08, 5) projected
  line L774 (304.255, -5) -> (301.08, -5) projected
  line L775 (304.255, -5) -> (304.255, -15) projected
  line L776 (301.08, -15) -> (304.255, -15) projected
  line L777 (301.08, -25) -> (301.08, -15) projected
  line L778 (304.255, -25) -> (301.08, -25) projected
  line L779 (304.255, -25) -> (304.255, -35) projected
  line L780 (301.08, -35) -> (304.255, -35) projected
  line L781 (301.08, -45) -> (301.08, -35) projected
  line L782 (304.255, -45) -> (301.08, -45) projected
  line L783 (304.255, -45) -> (304.255, -55) projected
  line L784 (301.08, -55) -> (304.255, -55) projected
  line L785 (301.08, -65) -> (301.08, -55) projected
  line L786 (304.255, -65) -> (301.08, -65) projected
  line L787 (304.255, -65) -> (304.255, -75) projected
  line L788 (301.08, -75) -> (304.255, -75) projected
  line L789 (301.08, -75) -> (301.08, -86.825) projected
  line L790 (301.08, -86.825) -> (306.08, -86.825) projected
  line L791 (306.08, -86.825) -> (306.08, -90) projected
  line L792 (306.08, -90) -> (316.08, -90) projected
  line L793 (316.08, -90) -> (316.08, -86.825) projected
  line L794 (316.08, -86.825) -> (326.08, -86.825) projected
  line L795 (326.08, -86.825) -> (326.08, -90) projected
  line L796 (326.08, -90) -> (336.08, -90) projected
  line L797 (336.08, -90) -> (336.08, -86.825) projected
  line L798 (336.08, -86.825) -> (346.08, -86.825) projected
  line L799 (346.08, -86.825) -> (346.08, -90) projected
  line L800 (346.08, -90) -> (356.08, -90) projected
  line L801 (356.08, -90) -> (356.08, -86.825) projected
  line L802 (356.08, -86.825) -> (366.08, -86.825) projected
  line L803 (366.08, -86.825) -> (366.08, -90) projected
  line L804 (366.08, -90) -> (376.08, -90) projected
  line L805 (376.08, -90) -> (376.08, -86.825) projected
  line L806 (376.08, -86.825) -> (386.08, -86.825) projected
  line L807 (386.08, -86.825) -> (386.08, -90) projected
  line L808 (386.08, -90) -> (396.08, -90) projected
  line L809 (396.08, -90) -> (396.08, -86.825) projected
  line L810 (396.08, -86.825) -> (406.08, -86.825) projected
  line L811 (406.08, -86.825) -> (406.08, -90) projected
  line L812 (406.08, -90) -> (416.08, -90) projected
  line L813 (416.08, -90) -> (416.08, -86.825) projected
  line L814 (416.08, -86.825) -> (421.08, -86.825) projected
  line L815 (421.08, -86.825) -> (421.08, -75) projected
  line L816 (421.08, -75) -> (417.905, -75) projected
  line L817 (417.905, -75) -> (417.905, -65) projected
  line L818 (417.905, -65) -> (421.08, -65) projected
  line L819 (421.08, -65) -> (421.08, -55) projected
  line L820 (421.08, -55) -> (417.905, -55) projected
  line L821 (417.905, -55) -> (417.905, -51.5) projected
  line L822 (417.905, -51.5) -> (415.905, -51.5) projected
  line L823 (415.905, -51.5) -> (415.905, -52.75) projected
  line L824 (415.905, -52.75) -> (413.405, -52.75) projected
  line L825 (413.405, -52.75) -> (413.405, -51.5) projected
  line L826 (413.405, -51.5) -> (407.08, -51.5) projected
  line L827 (407.08, -51.5) -> (407.08, -48.5) projected
  line L828 (407.08, -48.5) -> (413.405, -48.5) projected
  line L829 (413.405, -48.5) -> (413.405, -47.25) projected
  line L830 (413.405, -47.25) -> (415.905, -47.25) projected
  line L831 (415.905, -47.25) -> (415.905, -48.5) projected
  circle A19 centre (384.0772, -27.4451) radius 3 projected
  circle A20 centre (338.0828, 54) radius 3 projected
  circle A21 centre (384.0772, 27.4451) radius 3 projected
  circle A22 centre (338.0828, -54) radius 3 projected
  circle A23 centre (346.08, 8.175) radius 11 projected
  line L832 (466.08, -207.185) -> (477.905, -207.185) projected
  line L833 (477.905, -207.185) -> (477.905, -205.36) projected
  line L834 (477.905, -205.36) -> (481.08, -205.36) projected
  line L835 (481.08, -205.36) -> (481.08, -195.36) projected
  line L836 (481.08, -195.36) -> (477.905, -195.36) projected
  line L837 (477.905, -195.36) -> (477.905, -185.36) projected
  line L838 (477.905, -185.36) -> (481.08, -185.36) projected
  line L839 (481.08, -185.36) -> (481.08, -175.36) projected
  line L840 (481.08, -175.36) -> (477.905, -175.36) projected
  line L841 (477.905, -175.36) -> (477.905, -165.36) projected
  line L842 (477.905, -165.36) -> (481.08, -165.36) projected
  line L843 (481.08, -165.36) -> (481.08, -155.36) projected
  line L844 (481.08, -155.36) -> (477.905, -155.36) projected
  line L845 (477.905, -155.36) -> (477.905, -145.36) projected
  line L846 (477.905, -145.36) -> (481.08, -145.36) projected
  line L847 (481.08, -145.36) -> (481.08, -135.36) projected
  line L848 (481.08, -135.36) -> (477.905, -135.36) projected
  line L849 (477.905, -135.36) -> (477.905, -125.36) projected
  line L850 (477.905, -125.36) -> (481.08, -125.36) projected
  line L851 (481.08, -125.36) -> (481.08, -115.36) projected
  line L852 (481.08, -115.36) -> (477.905, -115.36) projected
  line L853 (477.905, -115.36) -> (477.905, -105.36) projected
  line L854 (477.905, -105.36) -> (481.08, -105.36) projected
  line L855 (481.08, -105.36) -> (481.08, -95.36) projected
  line L856 (481.08, -95.36) -> (477.905, -95.36) projected
  line L857 (477.905, -95.36) -> (477.905, -93.535) projected
  line L858 (477.905, -93.535) -> (466.08, -93.535) projected
  line L859 (466.08, -93.535) -> (466.08, -90.36) projected
  line L860 (466.08, -90.36) -> (456.08, -90.36) projected
  line L861 (456.08, -90.36) -> (456.08, -93.535) projected
  line L862 (456.08, -93.535) -> (446.08, -93.535) projected
  line L863 (446.08, -93.535) -> (446.08, -90.36) projected
  line L864 (446.08, -90.36) -> (436.08, -90.36) projected
  line L865 (436.08, -90.36) -> (436.08, -93.535) projected
  line L866 (436.08, -93.535) -> (426.08, -93.535) projected
  line L867 (426.08, -93.535) -> (426.08, -90.36) projected
  line L868 (426.08, -90.36) -> (416.08, -90.36) projected
  line L869 (416.08, -90.36) -> (416.08, -93.535) projected
  line L870 (416.08, -93.535) -> (406.08, -93.535) projected
  line L871 (406.08, -93.535) -> (406.08, -90.36) projected
  line L872 (406.08, -90.36) -> (396.08, -90.36) projected
  line L873 (396.08, -90.36) -> (396.08, -93.535) projected
  line L874 (396.08, -93.535) -> (386.08, -93.535) projected
  line L875 (386.08, -93.535) -> (386.08, -90.36) projected
  line L876 (386.08, -90.36) -> (376.08, -90.36) projected
  line L877 (376.08, -90.36) -> (376.08, -93.535) projected
  line L878 (376.08, -93.535) -> (366.08, -93.535) projected
  line L879 (366.08, -93.535) -> (366.08, -90.36) projected
  line L880 (366.08, -90.36) -> (356.08, -90.36) projected
  line L881 (356.08, -90.36) -> (356.08, -93.535) projected
  line L882 (356.08, -93.535) -> (346.08, -93.535) projected
  line L883 (346.08, -93.535) -> (346.08, -90.36) projected
  line L884 (346.08, -90.36) -> (336.08, -90.36) projected
  line L885 (336.08, -90.36) -> (336.08, -93.535) projected
  line L886 (336.08, -93.535) -> (326.08, -93.535) projected
  line L887 (326.08, -93.535) -> (326.08, -90.36) projected
  line L888 (326.08, -90.36) -> (316.08, -90.36) projected
  line L889 (316.08, -90.36) -> (316.08, -93.535) projected
  line L890 (316.08, -93.535) -> (304.255, -93.535) projected
  line L891 (304.255, -93.535) -> (304.255, -95.36) projected
  line L892 (304.255, -95.36) -> (301.08, -95.36) projected
  line L893 (301.08, -95.36) -> (301.08, -105.36) projected
  line L894 (301.08, -105.36) -> (304.255, -105.36) projected
  line L895 (304.255, -105.36) -> (304.255, -115.36) projected
  line L896 (304.255, -115.36) -> (301.08, -115.36) projected
  line L897 (301.08, -115.36) -> (301.08, -125.36) projected
  line L898 (301.08, -125.36) -> (304.255, -125.36) projected
  line L899 (304.255, -125.36) -> (304.255, -135.36) projected
  line L900 (304.255, -135.36) -> (301.08, -135.36) projected
  line L901 (301.08, -135.36) -> (301.08, -145.36) projected
  line L902 (301.08, -145.36) -> (304.255, -145.36) projected
  line L903 (304.255, -145.36) -> (304.255, -155.36) projected
  line L904 (304.255, -155.36) -> (301.08, -155.36) projected
  line L905 (301.08, -155.36) -> (301.08, -165.36) projected
  line L906 (301.08, -165.36) -> (304.255, -165.36) projected
  line L907 (304.255, -165.36) -> (304.255, -175.36) projected
  line L908 (304.255, -175.36) -> (301.08, -175.36) projected
  line L909 (301.08, -175.36) -> (301.08, -185.36) projected
  line L910 (301.08, -185.36) -> (304.255, -185.36) projected
  line L911 (304.255, -185.36) -> (304.255, -195.36) projected
  line L912 (304.255, -195.36) -> (301.08, -195.36) projected
  line L913 (301.08, -195.36) -> (301.08, -205.36) projected
  line L914 (301.08, -205.36) -> (304.255, -205.36) projected
  line L915 (304.255, -205.36) -> (304.255, -207.185) projected
  line L916 (304.255, -207.185) -> (316.08, -207.185) projected
  line L917 (316.08, -207.185) -> (316.08, -210.36) projected
  line L918 (316.08, -210.36) -> (326.08, -210.36) projected
  line L919 (326.08, -210.36) -> (326.08, -207.185) projected
  line L920 (326.08, -207.185) -> (336.08, -207.185) projected
  line L921 (336.08, -207.185) -> (336.08, -210.36) projected
  line L922 (336.08, -210.36) -> (346.08, -210.36) projected
  line L923 (346.08, -210.36) -> (346.08, -207.185) projected
  line L924 (346.08, -207.185) -> (356.08, -207.185) projected
  line L925 (356.08, -207.185) -> (356.08, -210.36) projected
  line L926 (356.08, -210.36) -> (366.08, -210.36) projected
  line L927 (366.08, -210.36) -> (366.08, -207.185) projected
  line L928 (366.08, -207.185) -> (376.08, -207.185) projected
  line L929 (376.08, -207.185) -> (376.08, -210.36) projected
  line L930 (376.08, -210.36) -> (386.08, -210.36) projected
  line L931 (386.08, -210.36) -> (386.08, -207.185) projected
  line L932 (386.08, -207.185) -> (396.08, -207.185) projected
  line L933 (396.08, -207.185) -> (396.08, -210.36) projected
  line L934 (396.08, -210.36) -> (406.08, -210.36) projected
  line L935 (406.08, -210.36) -> (406.08, -207.185) projected
  line L936 (406.08, -207.185) -> (416.08, -207.185) projected
  line L937 (416.08, -207.185) -> (416.08, -210.36) projected
  line L938 (416.08, -210.36) -> (426.08, -210.36) projected
  line L939 (426.08, -210.36) -> (426.08, -207.185) projected
  line L940 (426.08, -207.185) -> (436.08, -207.185) projected
  line L941 (436.08, -207.185) -> (436.08, -210.36) projected
  line L942 (436.08, -210.36) -> (446.08, -210.36) projected
  line L943 (446.08, -210.36) -> (446.08, -207.185) projected
  line L944 (446.08, -207.185) -> (456.08, -207.185) projected
  line L945 (456.08, -207.185) -> (456.08, -210.36) projected
  line L946 (456.08, -210.36) -> (466.08, -210.36) projected
  line L947 (466.08, -210.36) -> (466.08, -207.185) projected
  line L948 (331.08, -106.56) -> (451.08, -106.56) projected
  line L949 (451.08, -106.56) -> (451.08, -194.16) projected
  line L950 (451.08, -194.16) -> (331.08, -194.16) projected
  line L951 (331.08, -194.16) -> (331.08, -106.56) projected
  circle A24 centre (533.716, -59.1479) radius 1.078 projected
  circle A25 centre (498.716, -59.1479) radius 1.078 projected
  line L952 (525.255, -13.335) -> (521.445, -13.335) projected
  line L953 (521.445, -13.335) -> (521.445, -1.905) projected
  line L954 (521.445, -1.905) -> (525.255, -1.905) projected
  line L955 (525.255, -1.905) -> (525.255, -13.335) projected
  circle A26 centre (519.54, -15.24) radius 1.078 projected
  circle A27 centre (527.16, 0) radius 1.078 projected
  circle A28 centre (527.16, -15.24) radius 1.078 projected
  circle A29 centre (519.54, 0) radius 1.078 projected
  line L956 (536.265, -48.5) -> (538.265, -48.5) projected
  line L957 (538.265, -48.5) -> (538.265, -45) projected
  line L958 (538.265, -45) -> (541.44, -45) projected
  line L959 (541.44, -45) -> (541.44, -35) projected
  line L960 (541.44, -35) -> (538.265, -35) projected
  line L961 (538.265, -35) -> (538.265, -25) projected
  line L962 (538.265, -25) -> (541.44, -25) projected
  line L963 (541.44, -25) -> (541.44, -15) projected
  line L964 (541.44, -15) -> (538.265, -15) projected
  line L965 (538.265, -15) -> (538.265, -5) projected
  line L966 (538.265, -5) -> (541.44, -5) projected
  line L967 (541.44, -5) -> (541.44, 5) projected
  line L968 (541.44, 5) -> (538.265, 5) projected
  line L969 (538.265, 5) -> (538.265, 15) projected
  line L970 (538.265, 15) -> (541.44, 15) projected
  line L971 (541.44, 15) -> (541.44, 25) projected
  line L972 (541.44, 25) -> (538.265, 25) projected
  line L973 (538.265, 25) -> (538.265, 35) projected
  line L974 (538.265, 35) -> (541.44, 35) projected
  line L975 (541.44, 35) -> (541.44, 45) projected
  line L976 (541.44, 45) -> (538.265, 45) projected
  line L977 (538.265, 45) -> (538.265, 48.5) projected
  line L978 (538.265, 48.5) -> (536.265, 48.5) projected
  line L979 (536.265, 48.5) -> (536.265, 47.25) projected
  line L980 (536.265, 47.25) -> (533.765, 47.25) projected
  line L981 (533.765, 47.25) -> (533.765, 48.5) projected
  line L982 (533.765, 48.5) -> (527.44, 48.5) projected
  line L983 (527.44, 48.5) -> (527.44, 51.5) projected
  line L984 (527.44, 51.5) -> (533.765, 51.5) projected
  line L985 (533.765, 51.5) -> (533.765, 52.75) projected
  line L986 (533.765, 52.75) -> (536.265, 52.75) projected
  line L987 (536.265, 52.75) -> (536.265, 51.5) projected
  line L988 (536.265, 51.5) -> (538.265, 51.5) projected
  line L989 (538.265, 51.5) -> (538.265, 55) projected
  line L990 (538.265, 55) -> (541.44, 55) projected
  line L991 (541.44, 55) -> (541.44, 65) projected
  line L992 (541.44, 65) -> (538.265, 65) projected
  line L993 (538.265, 65) -> (538.265, 75) projected
  line L994 (538.265, 75) -> (541.44, 75) projected
  line L995 (541.44, 75) -> (541.44, 86.825) projected
  line L996 (536.44, 86.825) -> (541.44, 86.825) projected
  line L997 (536.44, 90) -> (536.44, 86.825) projected
  line L998 (526.44, 90) -> (536.44, 90) projected
  line L999 (526.44, 86.825) -> (526.44, 90) projected
  line L1000 (526.44, 86.825) -> (516.44, 86.825) projected
  line L1001 (516.44, 90) -> (516.44, 86.825) projected
  line L1002 (506.44, 90) -> (516.44, 90) projected
  line L1003 (506.44, 86.825) -> (506.44, 90) projected
  line L1004 (506.44, 86.825) -> (496.44, 86.825) projected
  line L1005 (496.44, 90) -> (496.44, 86.825) projected
  line L1006 (486.44, 90) -> (496.44, 90) projected
  line L1007 (486.44, 86.825) -> (486.44, 90) projected
  line L1008 (486.44, 86.825) -> (476.44, 86.825) projected
  line L1009 (476.44, 90) -> (476.44, 86.825) projected
  line L1010 (466.44, 90) -> (476.44, 90) projected
  line L1011 (466.44, 86.825) -> (466.44, 90) projected
  line L1012 (466.44, 86.825) -> (456.44, 86.825) projected
  line L1013 (456.44, 90) -> (456.44, 86.825) projected
  line L1014 (446.44, 90) -> (456.44, 90) projected
  line L1015 (446.44, 86.825) -> (446.44, 90) projected
  line L1016 (446.44, 86.825) -> (436.44, 86.825) projected
  line L1017 (436.44, 90) -> (436.44, 86.825) projected
  line L1018 (426.44, 90) -> (436.44, 90) projected
  line L1019 (426.44, 86.825) -> (426.44, 90) projected
  line L1020 (426.44, 86.825) -> (421.44, 86.825) projected
  line L1021 (421.44, 75) -> (421.44, 86.825) projected
  line L1022 (424.615, 75) -> (421.44, 75) projected
  line L1023 (424.615, 75) -> (424.615, 65) projected
  line L1024 (421.44, 65) -> (424.615, 65) projected
  line L1025 (421.44, 55) -> (421.44, 65) projected
  line L1026 (424.615, 55) -> (421.44, 55) projected
  line L1027 (424.615, 55) -> (424.615, 45) projected
  line L1028 (421.44, 45) -> (424.615, 45) projected
  line L1029 (421.44, 35) -> (421.44, 45) projected
  line L1030 (424.615, 35) -> (421.44, 35) projected
  line L1031 (424.615, 35) -> (424.615, 25) projected
  line L1032 (421.44, 25) -> (424.615, 25) projected
  line L1033 (421.44, 15) -> (421.44, 25) projected
  line L1034 (424.615, 15) -> (421.44, 15) projected
  line L1035 (424.615, 15) -> (424.615, 5) projected
  line L1036 (421.44, 5) -> (424.615, 5) projected
  line L1037 (421.44, -5) -> (421.44, 5) projected
  line L1038 (424.615, -5) -> (421.44, -5) projected
  line L1039 (424.615, -5) -> (424.615, -15) projected
  line L1040 (421.44, -15) -> (424.615, -15) projected
  line L1041 (421.44, -25) -> (421.44, -15) projected
  line L1042 (424.615, -25) -> (421.44, -25) projected
  line L1043 (424.615, -25) -> (424.615, -35) projected